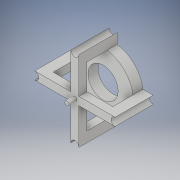
# Autodesk Inventor part: CheckValveValve1.0
Saved by Autodesk Inventor 2019 (Build 230136000, 136)
## iProperties
Created: 2019-04-04
Part Number: CheckValveValve1.0
Material: Generic
Document SubType Name: Modeling
Designer: Kepler
Density: 1 g/cm^3
Appearance: Default
Author: Kepler
Autodesk Inventor part; units mm, degrees
ref_plane "YZ Plane" through (0, 0, 0) normal (1, 0, 0) x (0, 1, 0)
ref_plane "XZ Plane" through (0, 0, 0) normal (0, 1, 0) x (-1, 0, 0)
ref_plane "XY Plane" through (0, 0, 0) normal (0, 0, 1) x (1, 0, 0)
sketch "Sketch1" plane through (0, 0, 0) normal (0, 0, 1) x (1, 0, 0)
  arc A0 (-2, 20) -> (2, 20) centre (0, 20) ccw
  arc A1 (20, 2) -> (20, -2) centre (20, 0) ccw
  arc A2 (2, -20) -> (-2, -20) centre (0, -20) ccw
  arc A3 (-20, -2) -> (-20, 2) centre (-20, 0) ccw
  circle A4 centre (0, 0) radius 7.5
  line L0 (-2, 20) -> (-2, 14.8661)
  line L1 (2, 20) -> (2, 14.8661)
  line L2 (20, 2) -> (14.8661, 2)
  line L3 (20, -2) -> (14.8661, -2)
  line L4 (2, -20) -> (2, -14.8661)
  line L5 (-2, -14.8661) -> (-2, -20)
  line L6 (-20, -2) -> (-14.8661, -2)
  line L7 (-20, 2) -> (-14.8661, 2)
  arc A5 (-14.8661, -2) -> (-2, -14.8661) centre (0, 0) ccw
  arc A6 (-2, 14.8661) -> (-14.8661, 2) centre (0, 0) ccw
  arc A7 (2, -14.8661) -> (14.8661, -2) centre (0, 0) ccw
  arc A8 (14.8661, 2) -> (2, 14.8661) centre (0, 0) ccw
  dimension "d0" = 4
  dimension "d1" = 4
  dimension "d2" = 4
  dimension "d3" = 4
  dimension "d5" = 15
  constraints: 16 end point, 16 point on circle, 9 centre point, 8 point on line, 3 tangent, 2 coincident, 2 parallel, 1 perpendicular, 1 vertical
  measures "d0" diameter of A0
  measures "d1" diameter of A1
  measures "d2" diameter of A2
  measures "d3" diameter of A3
  measures "d5" diameter of A4
extrude "Extrusion1" add sketch "Sketch1" along normal blind 5
sketch "Sketch2" plane through (0, 0, 0) normal (0, 0, -1) x (-1, 0, 0)
  circle A0 centre (0, 0) radius 8.5
  circle A1 centre (0, 0) radius 14
  dimension "d8" = 17
  dimension "d9" = 28
  constraints: 2 centre point, 2 coincident
  measures "d8" diameter of A0
  measures "d9" diameter of A1
extrude "Extrusion2" cut sketch "Sketch2" against normal blind 1
sketch "Sketch3" plane through (0, 0, 5) normal (0, 0, 1) x (1, 0, 0)
  line L0 (2, -14.8661) -> (2, -20) projected
  arc A0 (-2, -14.8661) -> (2, -14.8661) centre (0, 0) ccw
  circle A1 centre (0, 0) radius 14 projected
  arc A2 (-14.8661, -2) -> (-2, -14.8661) centre (0, 0) ccw projected
  arc A3 (-14.8661, 2) -> (-14.8661, -2) centre (0, 0) ccw
  arc A4 (-2, 14.8661) -> (-14.8661, 2) centre (0, 0) ccw projected
  arc A5 (2, 14.8661) -> (-2, 14.8661) centre (0, 0) ccw
  line L1 (20, -2) -> (14.8661, -2) projected
  arc A6 (14.8661, 2) -> (2, 14.8661) centre (0, 0) ccw projected
  arc A7 (14.8661, -2) -> (14.8661, 2) centre (0, 0) ccw
  line L2 (-2, 14.8661) -> (-2, 20) projected
  arc A8 (-2, 20) -> (2, 20) centre (0, 20) ccw projected
  arc A9 (-2, 20) -> (2, 20) centre (0, 20) ccw
  arc A10 (20, 2) -> (20, -2) centre (20, 0) ccw projected
  arc A11 (20, 2) -> (20, -2) centre (20, 0) ccw
  line L3 (-2, -20) -> (-2, -14.8661) projected
  arc A12 (2, -20) -> (-2, -20) centre (0, -20) ccw
  arc A13 (-20, -2) -> (-20, 2) centre (-20, 0) ccw projected
  arc A14 (-20, -2) -> (-20, 2) centre (-20, 0) ccw
  line L4 (-2, 14.8661) -> (-2, 20)
  line L5 (2, 20) -> (2, 14.8661) projected
  line L6 (2, 20) -> (2, 14.8661)
  line L7 (-20, 2) -> (-14.8661, 2)
  line L8 (-2, -20) -> (-2, -14.8661)
  arc A15 (2, -20) -> (-2, -20) centre (0, -20) ccw projected
  line L9 (2, -14.8661) -> (2, -20)
  line L10 (20, -2) -> (14.8661, -2)
  line L11 (14.8661, 2) -> (20, 2) projected
  line L12 (20, 2) -> (14.8661, 2)
  line L13 (-14.8661, -2) -> (-20, -2) projected
  line L14 (-20, -2) -> (-14.8661, -2)
  constraints: 18 point on circle, 16 end point, 8 centre point, 7 tangent, 6 collinear, 5 coincident, 1 concentric, 1 horizontal
ref_plane "Work Plane1" through (0, 0, 15) normal (0, 0, 1) x (1, 0, 0)
sketch "Sketch4" plane through (0, 0, 15) normal (0, 0, 1) x (1, 0, 0)
  line L0 (2, 14.8661) -> (2, 20) projected
  line L1 (2, 14.8661) -> (2, 2)
  line L2 (14.8661, 2) -> (20, 2) projected
  line L3 (2, 2) -> (14.8661, 2)
  arc A0 (14.8661, -2) -> (14.8661, 2) centre (0, 0) ccw projected
  line L4 (14.8661, -2) -> (2, -2)
  arc A1 (-2, -14.8661) -> (2, -14.8661) centre (0, 0) ccw projected
  line L5 (2, -2) -> (2, -14.8661)
  line L6 (-2, -14.8661) -> (-2, -2)
  arc A2 (-14.8661, -2) -> (-2, -14.8661) centre (0, 0) ccw projected
  line L7 (-2, -2) -> (-14.8661, -2)
  line L8 (-14.8661, 2) -> (-20, 2) projected
  line L9 (-14.8661, 2) -> (-2, 2)
  line L10 (-2, 20) -> (-2, 14.8661) projected
  line L11 (-2, 2) -> (-2, 14.8661)
  arc A3 (2, 14.8661) -> (-2, 14.8661) centre (0, 0) ccw projected
  arc A4 (2, 14.8661) -> (-2, 14.8661) centre (0, 0) ccw
  arc A5 (2, -14.8661) -> (14.8661, -2) centre (0, 0) ccw projected
  arc A6 (14.8661, -2) -> (14.8661, 2) centre (0, 0) ccw
  arc A7 (-2, -14.8661) -> (2, -14.8661) centre (0, 0) ccw
  arc A8 (-14.8661, 2) -> (-14.8661, -2) centre (0, 0) ccw
  constraints: 16 end point, 8 point on circle, 5 perpendicular, 4 centre point, 4 coincident, 2 horizontal, 1 vertical
extrude "Extrusion4" add sketch "Sketch3" along normal blind 14 contours L0 A12 L3 A0 | A3 L13 A13 L7 | A5 L2 A8 L5 | L1 A7 L11 A10
extrude "Extrusion5" add sketch "Sketch4" along normal blind 4 contours L1 L3 A0 L4 L5 A1 L6 L7 A8 L9 L11 A3
sketch "Sketch5" plane through (0, 0, 19) normal (0, 0, 1) x (1, 0, 0)
  circle A0 centre (0, 0) radius 1
  dimension "d18" = 2
  constraints: 1 centre point, 1 coincident
  measures "d18" diameter of A0
extrude "Extrusion6" add sketch "Sketch5" along normal blind 4
body "Solid1"
